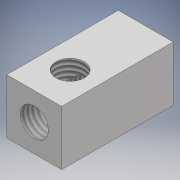
# Autodesk Inventor part: M3_cube_standoff
Saved by Autodesk Inventor 2018 (Build 220112000, 112)
## iProperties
Created: 2018-05-21
Part Number: M3_cube_standoff
Material: Generic
Document SubType Name: Modeling
Designer: etd
Density: 1 g/cm^3
Appearance: Default
square_width: 5,800 mm
height: 11,800 mm
central_hole_to_side: 2,900 mm
side_hole_to_side_long: 8,000 mm
side_hole_to_side_short: 3,800 mm
side_hole_to_side_intermediate: 2,900 mm
Author: etd
Autodesk Inventor part; units mm, degrees
ref_plane "YZ Plane" through (0, 0, 0) normal (1, 0, 0) x (0, 1, 0)
ref_plane "XZ Plane" through (0, 0, 0) normal (0, 1, 0) x (-1, 0, 0)
ref_plane "XY Plane" through (0, 0, 0) normal (0, 0, 1) x (1, 0, 0)
sketch "Sketch1" plane through (0, 0, 0) normal (0, 1, 0) x (-1, 0, 0)
  line L0 (-2.9, 2.9) -> (2.9, 2.9)
  line L1 (2.9, 2.9) -> (2.9, -2.9)
  line L2 (2.9, -2.9) -> (-2.9, -2.9)
  line L3 (-2.9, -2.9) -> (-2.9, 2.9)
  line L4 (-2.9, 2.9) -> (2.9, -2.9) construction
  line L5 (2.9, 2.9) -> (-2.9, -2.9) construction
  point P0 (0, 0)
  point P1 (0, 0)
  dimension "d0" = 5.8
  constraints: 12 end point, 2 midpoint, 2 parallel, 2 perpendicular, 1 coincident, 1 horizontal
  measures "d0" distance of L1.end L2.end
extrude "Extrusion1" add sketch "Sketch1" along normal blind 11.8
hole "Hole1" at (0, 0, 0) direction (0, 1, 0) diameter 3 end through all
thread "Thread1" size "M3x0.5" class "6H" standard "ANSI Metric M Profile" full length
sketch "Sketch2" plane through (-2.9, 0, 2.9) normal (0, 0, 1) x (1, 0, 0)
  line L0 (5.8, 0) -> (0, 0) projected
  line L1 (5.8, 0) -> (5.8, 11.8) projected
  line L2 (0, 11.8) -> (5.8, 11.8) projected
  line L3 (0, 0) -> (0, 11.8) projected
  line L4 (2.9, 0) -> (2.9, 3.8) construction
  dimension "d12" = 3.8
  constraints: 2 end point, 1 coincident, 1 vertical
  measures "d12" distance of L4.start L4.end
hole "Hole2" at (0, 3.8, 2.9) direction (0, 0, -1) diameter 3 end through all
thread "Thread2" size "M3x0.5" class "6H" standard "ANSI Metric M Profile" full length
equation "\"square_width\" = d0"
equation "\"height\" = d1"
equation "\"side_hole_to_side_short\" = d12"
equation "\"side_hole_to_side_long\" = height - side_hole_to_side_short"
equation "\"side_hole_to_side_intermediate\" = 0.5 * square_width"
equation "\"central_hole_to_side\" = 0.5 * square_width"
equation "\"d1\" = 11.8"
body "Solid1"
